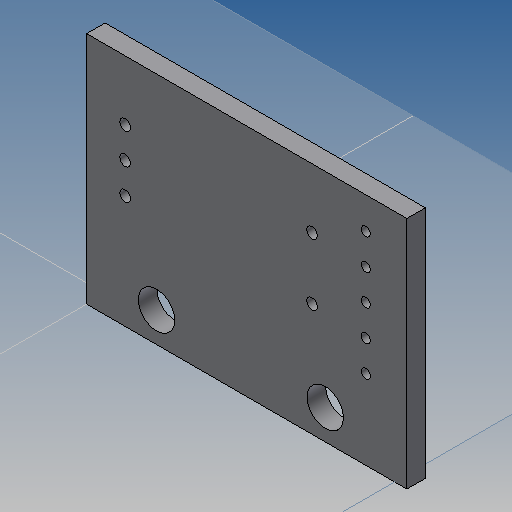
# Autodesk Inventor part: pcb
Saved by Autodesk Inventor 2019 (Build 230136000, 136)
## iProperties
Created: 2015-11-19
Part Number: pcb
Material: Allgemein
Document SubType Name: Modeling
Designer: Tom
Density: 1 g/cm^3
Appearance: Vorgabe
Mass: 0.748413 g
Surface Area: 11.8985 cm^2
Volume: 0.748413 cm^3
Author: Tom
Autodesk Inventor part; units mm, degrees
ref_plane "YZ Plane" through (0, 0, 0) normal (1, 0, 0) x (0, 1, 0)
ref_plane "XZ Plane" through (0, 0, 0) normal (0, 1, 0) x (-1, 0, 0)
ref_plane "XY Plane" through (0, 0, 0) normal (0, 0, 1) x (1, 0, 0)
sketch "Sketch1" plane through (0, 0, 0) normal (0, 0, 1) x (1, 0, 0)
  line L0 (0, 0) -> (26.416, 0)
  line L1 (26.416, 0) -> (26.416, 19.3294)
  line L2 (26.416, 19.3294) -> (0, 19.3294)
  line L3 (0, 19.3294) -> (0, 0)
  circle A0 centre (5.7658, 2.4638) radius 1.5
  circle A1 centre (19.685, 2.4638) radius 1.5
  line L4 (21.8186, 5.2832) -> (24.2316, 5.2832)
  line L5 (24.2316, 5.2832) -> (24.2316, 17.9832)
  line L6 (24.2316, 17.9832) -> (21.8186, 17.9832)
  line L7 (21.8186, 17.9832) -> (21.8186, 5.2832)
  circle A2 centre (23.0251, 6.5532) radius 0.381
  circle A3 centre (23.0251, 9.0932) radius 0.381
  circle A4 centre (23.0251, 11.6332) radius 0.381
  circle A5 centre (23.0251, 14.1732) radius 0.381
  circle A6 centre (23.0251, 16.7132) radius 0.381
  circle A7 centre (3.175, 14.4018) radius 0.4445
  circle A8 centre (3.175, 11.8618) radius 0.4445
  circle A9 centre (3.175, 9.3218) radius 0.4445
  circle A10 centre (18.593, 9.3218) radius 0.4445 projected
  dimension "d0" = 26.416
  dimension "d1" = 19.3294
  dimension "d2" = 3
  dimension "d3" = 3
  dimension "d4" = 5.7658
  dimension "d5" = 2.4638
  dimension "d6" = 13.9192
  dimension "d7" = 6.731
  dimension "d8" = 2.413
  dimension "d9" = 12.7
  dimension "d10" = 5.2832
  dimension "d11" = 2.1844
  dimension "d12" = 1.27
  dimension "d14" = 2.54
  dimension "d15" = 2.54
  dimension "d16" = 2.54
  dimension "d18" = 1.2065
  dimension "d19" = 2.54
  dimension "d20" = 0.762
  dimension "d21" = 0.762
  dimension "d22" = 0.762
  dimension "d23" = 0.762
  dimension "d24" = 0.762
  dimension "d25" = 0.889
  dimension "d26" = 0.889
  dimension "d27" = 0.889
  dimension "d28" = 4.9276
  dimension "d29" = 2.54
  dimension "d30" = 2.54
  dimension "d31" = 3.175
  constraints: 16 end point, 10 centre point, 6 vertical alignment, 5 coincident, 4 parallel, 2 horizontal, 2 perpendicular, 1 horizontal alignment
  measures "d0" distance of L2.end L1.end
  measures "d1" distance of L1.end L0.end
  measures "d2" diameter of A0
  measures "d3" diameter of A1
  measures "d4" distance from line of L3 A0.centre
  measures "d5" distance from line of L0 A0.centre
  measures "d6" distance of A1.centre A0.centre
  measures "d7" distance from line of L1 A1.centre
  measures "d8" distance of L6.end L5.end
  measures "d9" distance of L5.end L4.end
  measures "d10" distance from line of L0.end L4
  measures "d11" horizontal distance of L1.end L5.end
  measures "d12" vertical distance of point (23.025, 6.553) L4.end
  measures "d14" distance of point (23.025, 11.633) point (23.025, 9.093)
  measures "d15" distance of point (23.025, 14.173) point (23.025, 11.633)
  measures "d16" distance of point (23.025, 16.713) point (23.025, 14.173)
  measures "d18" distance from line of L7 point (23.025, 16.713)
  measures "d19" distance of point (23.025, 9.093) point (23.025, 6.553)
  measures "d20" diameter of A2
  measures "d21" diameter of A3
  measures "d22" diameter of A4
  measures "d23" diameter of A5
  measures "d24" diameter of A6
  measures "d25" diameter of A7
  measures "d26" diameter of A8
  measures "d27" diameter of A9
  measures "d28" vertical distance of L2.end A7.centre
  measures "d29" distance of A8.centre A7.centre
  measures "d30" distance of A9.centre A8.centre
  measures "d31" distance from line of L3 A7.centre
extrude "Extrusion1" add sketch "Sketch1" along normal blind 1.524 contours L3 L2 L1 L0 | L7 L6 L5 L4 | A10
sketch "Sketch3" plane through (0, 0, 1.524) normal (0, 0, 1) x (1, 0, 0)
  arc A0 (18.9807, 14.6193) -> (18.7439, 13.9837) centre (18.593, 14.4018) ccw projected
  circle A1 centre (18.593, 9.3218) radius 0.4445 projected
hole "Hole1" at (18.593, 14.4018, 1.524) at (18.593, 9.3218, 1.524) direction (0, 0, -1) diameter 0.889 end through all
equation "\"d18\" = 0.5 * d8"
equation "\"d26\" = d25"
equation "\"d27\" = d25"
body "Solid1"
